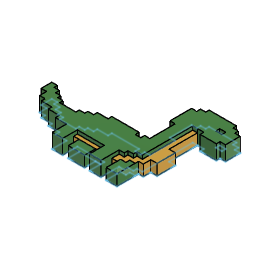
DinoKeychain (Autodesk Fusion 360 design; units mm, degrees)
Autodesk Fusion 360 part; units mm, degrees
sketch "Dino" plane through (0, 0, 0) normal (0, 0, 1) x (1, 0, 0)
  line L0 (-25.8333, -18.1173) -> (-25.8333, -25.4727)
  line L1 (-25.8333, -25.4727) -> (-22.0613, -25.4727)
  line L2 (-22.0613, -25.4727) -> (-22.0613, -30.282)
  line L3 (-22.0613, -30.282) -> (-18.2893, -30.282)
  line L4 (-18.2893, -30.282) -> (-18.2893, -32.9224)
  line L5 (-18.2893, -32.9224) -> (-10.9339, -32.9224)
  line L6 (-10.9339, -32.9224) -> (-10.9339, -35.3742)
  line L7 (-10.9339, -35.3742) -> (-3.3899, -35.3742)
  line L8 (-3.3899, -35.3742) -> (-3.3899, -38.0146)
  line L9 (-3.3899, -38.0146) -> (4.2484, -38.0146)
  line L10 (4.2484, -38.0146) -> (4.2484, -47.9161)
  line L11 (4.2484, -47.9161) -> (11.5095, -47.9161)
  line L12 (11.5095, -47.9161) -> (11.5095, -40.3721)
  line L13 (11.5095, -40.3721) -> (15.2815, -40.3721)
  line L14 (15.2815, -40.3721) -> (15.2815, -47.9161)
  line L15 (15.2815, -47.9161) -> (26.5975, -47.9161)
  line L16 (26.5975, -40.3721) -> (30.0866, -40.3721)
  line L17 (30.0866, -40.3721) -> (30.0866, -47.9161)
  line L18 (30.0866, -47.9161) -> (37.9135, -47.9161)
  line L19 (37.9135, -47.9161) -> (37.9135, -40.3721)
  line L20 (37.9135, -40.3721) -> (41.4969, -40.3721)
  line L21 (41.4969, -40.3721) -> (41.4969, -47.9161)
  line L22 (41.4969, -47.9161) -> (48.9466, -47.9161)
  line L23 (48.9466, -47.9161) -> (48.9466, -33.0167)
  line L24 (48.9466, -33.0167) -> (52.2471, -33.0167)
  line L25 (52.2471, -33.0167) -> (52.2471, -27.8302)
  line L26 (52.2471, -27.8302) -> (56.5849, -27.8302)
  line L27 (56.5849, -27.8302) -> (56.5849, -15.194)
  line L28 (56.5849, -15.194) -> (52.2471, -15.194)
  line L29 (52.2471, -15.194) -> (52.2471, 4.4204)
  line L30 (52.2471, 4.4204) -> (56.5849, 4.4204)
  line L31 (56.5849, 4.4204) -> (56.5849, 1.8743)
  line L32 (56.5849, 1.8743) -> (67.8065, 1.8743)
  line L33 (67.8065, 1.8743) -> (67.8065, 4.4204)
  line L34 (67.8065, 4.4204) -> (71.5785, 4.4204)
  line L35 (71.5785, 4.4204) -> (71.5785, 14.6048)
  line L36 (71.5785, 14.6048) -> (67.8065, 14.6048)
  line L37 (67.8065, 14.6048) -> (67.8065, 17.1509)
  line L38 (67.8065, 17.1509) -> (64.1289, 17.1509)
  line L39 (64.1289, 17.1509) -> (64.1289, 19.5084)
  line L40 (64.1289, 19.5084) -> (45.1746, 19.5084)
  line L41 (45.1746, 19.5084) -> (45.1746, 17.1509)
  line L42 (45.1746, 17.1509) -> (41.6855, 17.1509)
  line L43 (41.6855, 17.1509) -> (41.6855, 14.5105)
  line L44 (41.6855, 14.5105) -> (38.1021, 14.5105)
  line L45 (38.1021, 14.5105) -> (38.1021, -0.4832)
  line L46 (38.1021, -0.4832) -> (41.6855, -0.4832)
  line L47 (41.6855, -0.4832) -> (41.6855, -17.9287)
  line L48 (41.6855, -17.9287) -> (38.1021, -17.9287)
  line L49 (38.1021, -17.9287) -> (38.1021, -20.5691)
  line L50 (38.1021, -20.5691) -> (34.2358, -20.5691)
  line L51 (34.2358, -20.5691) -> (34.2358, -17.9287)
  line L52 (34.2358, -17.9287) -> (15.4701, -17.9287)
  line L53 (15.4701, -17.9287) -> (15.4701, -20.5691)
  line L54 (15.4701, -20.5691) -> (8.0204, -20.5691)
  line L55 (8.0204, -20.5691) -> (8.0204, -23.1152)
  line L56 (8.0204, -23.1152) -> (4.0598, -23.1152)
  line L57 (4.0598, -23.1152) -> (4.0598, -25.2841)
  line L58 (4.0598, -25.2841) -> (0.2878, -25.2841)
  line L59 (0.2878, -25.2841) -> (0.2878, -27.6416)
  line L60 (0.2878, -27.6416) -> (-10.8396, -27.6416)
  line L61 (-10.8396, -27.6416) -> (-10.8396, -25.2841)
  line L62 (-10.8396, -25.2841) -> (-14.5173, -25.2841)
  line L63 (-14.5173, -25.2841) -> (-14.5173, -23.1152)
  line L64 (-14.5173, -23.1152) -> (-18.195, -23.1152)
  line L65 (-18.195, -23.1152) -> (-18.195, -20.3805)
  line L66 (-18.195, -20.3805) -> (-21.967, -20.3805)
  line L67 (-25.8333, -18.1173) -> (-22.002, -18.1173)
  line L68 (-22.002, -18.1173) -> (-21.967, -20.3805)
  line L69 (11.5095, -40.3721) -> (11.5095, -37.7886)
  line L70 (11.5095, -37.7886) -> (30.0797, -37.7886)
  line L71 (30.0797, -37.7886) -> (30.0866, -40.3721)
  line L72 (30.0866, -40.3721) -> (26.5975, -40.3721)
  line L73 (37.9135, -40.3721) -> (37.9135, -35.4027)
  line L74 (37.9135, -35.4027) -> (41.4793, -35.4027)
  line L75 (41.4793, -35.4027) -> (41.4793, -32.8357)
  line L76 (41.4793, -32.8357) -> (45.2799, -32.8357)
  line L77 (45.2799, -32.8357) -> (45.2799, -30.4315)
  line L78 (45.2799, -30.4315) -> (49.0411, -30.4315)
  line L79 (49.0411, -30.4315) -> (49.0411, 4.3785)
  line L80 (49.0411, 4.3785) -> (52.2471, 4.4204)
  line L81 (59.9748, 12.022) -> (59.9748, 9.3751)
  line L82 (59.9748, 9.3751) -> (64.1657, 9.3751)
  line L83 (64.1657, 9.3751) -> (64.1657, 12.0124)
  line L84 (64.1657, 12.0124) -> (59.9748, 12.022)
  line L85 (15.2815, -40.3721) -> (26.5975, -40.3721)
  line L86 (26.5975, -45.2558) -> (26.5975, -47.9161)
  line L87 (26.5975, -45.2558) -> (26.5975, -40.3721)
  line L88 (41.4969, -40.3721) -> (41.4969, -38)
  line L89 (41.4969, -38) -> (45.2217, -38)
  line L90 (45.2217, -38) -> (45.2217, -35.3158)
  line L91 (45.2217, -35.3158) -> (48.9466, -35.3158)
  constraint vertical L0
  constraint perpendicular L0 L1
  constraint perpendicular L1 L2
  constraint perpendicular L2 L3
  constraint perpendicular L3 L4
  constraint perpendicular L4 L5
  constraint perpendicular L5 L6
  constraint perpendicular L6 L7
  constraint perpendicular L7 L8
  constraint perpendicular L8 L9
  constraint perpendicular L7 L10
  constraint perpendicular L10 L11
  constraint perpendicular L11 L12
  constraint perpendicular L12 L13
  constraint perpendicular L13 L14
  constraint perpendicular L14 L15
  constraint perpendicular L14 L16
  constraint perpendicular L16 L17
  constraint perpendicular L17 L18
  constraint perpendicular L18 L19
  constraint perpendicular L19 L20
  constraint perpendicular L20 L21
  constraint perpendicular L21 L22
  constraint perpendicular L22 L23
  constraint perpendicular L23 L24
  constraint perpendicular L24 L25
  constraint perpendicular L25 L26
  constraint perpendicular L26 L27
  constraint perpendicular L27 L28
  constraint perpendicular L28 L29
  constraint perpendicular L29 L30
  constraint perpendicular L30 L31
  constraint perpendicular L31 L32
  constraint perpendicular L32 L33
  constraint perpendicular L33 L34
  constraint perpendicular L34 L35
  constraint perpendicular L35 L36
  constraint perpendicular L36 L37
  constraint perpendicular L37 L38
  constraint perpendicular L38 L39
  constraint perpendicular L39 L40
  constraint perpendicular L40 L41
  constraint perpendicular L41 L42
  constraint perpendicular L42 L43
  constraint perpendicular L43 L44
  constraint perpendicular L44 L45
  constraint perpendicular L45 L46
  constraint perpendicular L46 L47
  constraint perpendicular L47 L48
  constraint perpendicular L46 L49
  constraint perpendicular L49 L50
  constraint perpendicular L50 L51
  constraint perpendicular L51 L52
  constraint perpendicular L52 L53
  constraint perpendicular L53 L54
  constraint perpendicular L54 L55
  constraint perpendicular L55 L56
  constraint perpendicular L56 L57
  constraint perpendicular L57 L58
  constraint perpendicular L58 L59
  constraint perpendicular L59 L60
  constraint perpendicular L60 L61
  constraint perpendicular L61 L62
  constraint perpendicular L62 L63
  constraint perpendicular L63 L64
  constraint perpendicular L64 L65
  constraint perpendicular L65 L66
  constraint perpendicular L0 L67
  constraint perpendicular L13 L69
  constraint perpendicular L69 L70
  constraint perpendicular L20 L73
  constraint perpendicular L73 L74
  constraint perpendicular L74 L75
  constraint perpendicular L75 L76
  constraint perpendicular L76 L77
  constraint perpendicular L77 L78
  constraint perpendicular L78 L79
  constraint vertical L81
  constraint perpendicular L81 L82
  constraint perpendicular L82 L83
  constraint perpendicular L15 L86
  constraint perpendicular L20 L88
  constraint perpendicular L21 L89
  constraint perpendicular L20 L90
  constraint coincident L23 L91.end
  constraint perpendicular L23 L91
extrude "Extrude18" add sketch "Dino" along normal blind 10 contours L0 L1 L2 L3 L4 L5 L6 L7 L8 L9 L10 L11 L12 L17 L18 L19 L30 L31 L32 L33 L34 L35 L36 L37 L38 L39 L40 L41 L42 L43 L44 L45 L46 L47 L48 L49 L50 L51 L52 L53 L54 L55 L56 L57 L58 L59 L60 L61 L62 L63 L64 L65 L66 L67 L68 L69 L70 L71 L73 L74 L75 L76 L77 L78 L79 L80
extrude "Extrude19" add sketch "Dino" along normal blind 7.5 contours L13 L16 L69 L70 L71 L72 L85 | L20 L23 L24 L25 L26 L27 L28 L29 L73 L74 L75 L76 L77 L78 L79 L80 L88 L89 L90 L91
extrude "Extrude20" add sketch "Dino" along normal blind 7.49 contours L14 L15 L85 L86 L87 | L21 L22 L23 L88 L89 L90 L91
extrude "Extrude21" cut sketch "Dino" along normal blind 0.01 contours L20 L23 L24 L25 L26 L27 L28 L29 L73 L74 L75 L76 L77 L78 L79 L80 L88 L89 L90 L91
named bodies: "DinoBody"
